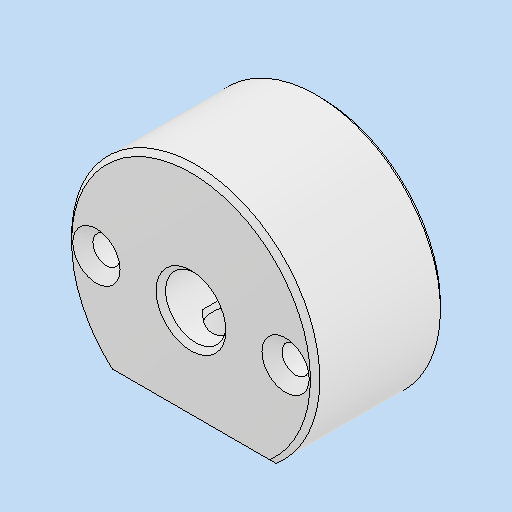
# Autodesk Inventor part: shaft-coupler-pla
Saved by Autodesk Inventor 2025 (Build 290162000, 162)
## iProperties
Created: 2025-05-28
Part Number: shaft-coupler-pla
Material: ABS Plastic
Document SubType Name: Modeling
Designer: kuzmin
Density: 1.06 g/cm^3
Appearance: Smooth - White
Author: kuzmin
Autodesk Inventor part; units mm, degrees
ref_plane "YZ Plane" through (0, 0, 0) normal (1, 0, 0) x (0, 1, 0)
ref_plane "XZ Plane" through (0, 0, 0) normal (0, 1, 0) x (-1, 0, 0)
ref_plane "XY Plane" through (0, 0, 0) normal (0, 0, 1) x (1, 0, 0)
sketch "Sketch1" plane through (0, 0, 0) normal (0, 0, 1) x (1, 0, 0)
  circle A0 centre (0, 0) radius 2.55
  circle A1 centre (0, 0) radius 10.5
  dimension "d0" = 21
  dimension "d1" = 5.1
  constraints: 2 centre point, 2 coincident
  measures "d0" diameter of A1
  measures "d1" diameter of A0
extrude "Extrusion1" add sketch "Sketch1" along normal blind 11
sketch "Sketch3" plane through (0, 0, 0) normal (0, 0, -1) x (-1, 0, 0)
  circle A0 centre (0, 0) radius 4.5
  dimension "d12" = 9
  constraints: 1 centre point, 1 coincident
  measures "d12" diameter of A0
extrude "Extrusion2" cut sketch "Sketch3" against normal blind 3
chamfer "Chamfer1" distance 1.93 angle 45 1 edges at (-2.55, 0, 3)
sketch "Sketch4" plane through (0, 0, 11) normal (0, 0, 1) x (1, 0, 0)
  line L0 (10, -8) -> (-10, -8)
  line L1 (-10, -8) -> (-10, -18)
  line L2 (-10, -18) -> (10, -18)
  line L3 (10, -18) -> (10, -8)
  point P0 (0, 0)
  point P1 (0, -8)
  dimension "d18" = 20
  dimension "d19" = 8
  dimension "d20" = 10
  constraints: 8 end point, 2 parallel, 1 horizontal, 1 midpoint, 1 perpendicular, 1 vertical alignment
  measures "d18" distance of L1.end L2.end
  measures "d19" distance from line of point (0, 0) L0
  measures "d20" distance of L2.end L0.start
extrude "Extrusion3" cut sketch "Sketch4" against normal through all
sketch "Sketch2" plane through (0, 0, 11) normal (0, 0, 1) x (1, 0, 0)
  circle A0 centre (0, 0) radius 8 construction
  point P0 (-8, 0)
  point P1 (8, 0)
  dimension "d4" = 16
  constraints: 2 horizontal alignment, 2 point on circle, 1 centre point, 1 coincident
  measures "d4" diameter of A0
hole "Hole1" at (-8, 0, 11) at (8, 0, 11) direction (0, 0, -1) diameter 2.3 end through all countersink diameter 4 countersink angle 90
sketch "Sketch5" plane through (0, 0, 0) normal (1, 0, 0) x (0, 1, 0)
  line L0 (-1, 7.2) -> (-12.4416, 7.2)
  line L1 (-8, 11) -> (-8, 0) projected
  line L2 (-8, 9.6) -> (-3, 9.6)
  line L3 (-3, 9.6) -> (-3, 9.2)
  line L4 (-3, 9.2) -> (-2, 9.2)
  line L5 (-2.55, 11) -> (-2.55, 4.93) projected
  line L6 (-2, 9.2) -> (-2, 7.2)
  line L7 (-8, 9.6) -> (-8, 7.2)
  line L8 (10.5, 11) -> (-8, 11) projected
  point P0 (0, 0)
  dimension "d23" = 4.8
  dimension "d24" = 4
  dimension "d25" = 5
  dimension "d27" = 1.4
  dimension "d28" = 1
  constraints: 12 end point, 4 point on line, 3 perpendicular, 2 horizontal
  measures "d23" diameter of L2 L0
  measures "d24" diameter of L4 L0
  measures "d25" distance of L2.start L2.end
  measures "d27" distance between parallel lines of L8 L2
  measures "d28" distance of L3.end L4.end
revolve "Revolution1" cut sketch "Sketch5" angle 360 about axis through (0, -1, 7.2) along (0, -1, 0) contours L0 L5 L4 L6 | L0 L1 L2 L3 L4 L5
chamfer "Chamfer2" distance 0.4 angle 45 8 edges at (0, 10.5, 11) (0, -8, 11) (0, 10.5, 0) (0, -8, 0) (4.5, 0, 0) (-8, 1.15, 0) (8, 1.15, 0) (-2.55, 0, 11)
body "Solid1"
